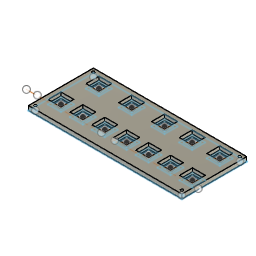
keyboard-holder (Autodesk Fusion 360 design; units mm, degrees)
Autodesk Fusion 360 part; units mm, degrees
sketch "Sketch1" plane through (0, 0, 0) normal (0, 0, 1) x (1, 0, 0)
  line L0 (-23.9041, 0) -> (63.45, 0) construction
  line L1 (78.95, 0) -> (176.0959, 0) construction
  line L2 (-1.45, -20) -> (177.05, -20)
  line L3 (177.05, -20) -> (177.05, 55.5)
  line L4 (177.05, 55.5) -> (-1.45, 55.5)
  line L5 (-1.45, 55.5) -> (-1.45, -20)
  line L6 (6.3, 0) -> (16.3, 0)
  line L7 (16.3, 0) -> (16.3, 10)
  line L8 (16.3, 10) -> (6.3, 10)
  line L9 (6.3, 10) -> (6.3, 0)
  line L10 (31.8, 0) -> (41.8, 0)
  line L11 (41.8, 0) -> (41.8, 10)
  line L12 (41.8, 10) -> (31.8, 10)
  line L13 (31.8, 10) -> (31.8, 0)
  line L14 (57.3, 0) -> (67.3, 0)
  line L15 (67.3, 0) -> (67.3, 10)
  line L16 (67.3, 10) -> (57.3, 10)
  line L17 (57.3, 10) -> (57.3, 0)
  line L18 (82.8, 0) -> (92.8, 0)
  line L19 (92.8, 0) -> (92.8, 10)
  line L20 (92.8, 10) -> (82.8, 10)
  line L21 (82.8, 10) -> (82.8, 0)
  line L22 (108.3, 0) -> (118.3, 0)
  line L23 (118.3, 0) -> (118.3, 10)
  line L24 (118.3, 10) -> (108.3, 10)
  line L25 (108.3, 10) -> (108.3, 0)
  line L26 (133.8, 0) -> (143.8, 0)
  line L27 (143.8, 0) -> (143.8, 10)
  line L28 (143.8, 10) -> (133.8, 10)
  line L29 (133.8, 10) -> (133.8, 0)
  line L30 (159.3, 0) -> (169.3, 0)
  line L31 (169.3, 0) -> (169.3, 10)
  line L32 (169.3, 10) -> (159.3, 10)
  line L33 (159.3, 10) -> (159.3, 0)
  line L34 (12.45, 48) -> (22.45, 48)
  line L35 (22.45, 48) -> (22.45, 38)
  line L36 (22.45, 38) -> (12.45, 38)
  line L37 (12.45, 38) -> (12.45, 48)
  line L38 (50.65, 48) -> (60.65, 48)
  line L39 (60.65, 48) -> (60.65, 38)
  line L40 (60.65, 38) -> (50.65, 38)
  line L41 (50.65, 38) -> (50.65, 48)
  line L42 (88.85, 48) -> (98.85, 48)
  line L43 (98.85, 48) -> (98.85, 38)
  line L44 (98.85, 38) -> (88.85, 38)
  line L45 (88.85, 38) -> (88.85, 48)
  line L46 (121, 48) -> (131, 48)
  line L47 (131, 48) -> (131, 38)
  line L48 (131, 38) -> (121, 38)
  line L49 (121, 38) -> (121, 48)
  line L50 (153.15, 48) -> (163.15, 48)
  line L51 (163.15, 48) -> (163.15, 38)
  line L52 (163.15, 38) -> (153.15, 38)
  line L53 (153.15, 38) -> (153.15, 48)
  line L54 (9.95, 50.5) -> (24.95, 50.5)
  line L55 (24.95, 50.5) -> (24.95, 35.5)
  line L56 (24.95, 35.5) -> (9.95, 35.5)
  line L57 (9.95, 35.5) -> (9.95, 50.5)
  line L58 (9.95, 50.5) -> (24.95, 35.5) construction
  line L59 (24.95, 50.5) -> (9.95, 35.5) construction
  line L60 (48.15, 50.5) -> (63.15, 50.5)
  line L61 (63.15, 50.5) -> (63.15, 35.5)
  line L62 (63.15, 35.5) -> (48.15, 35.5)
  line L63 (48.15, 35.5) -> (48.15, 50.5)
  line L64 (48.15, 50.5) -> (63.15, 35.5) construction
  line L65 (63.15, 50.5) -> (48.15, 35.5) construction
  line L66 (86.35, 50.5) -> (101.35, 50.5)
  line L67 (101.35, 50.5) -> (101.35, 35.5)
  line L68 (101.35, 35.5) -> (86.35, 35.5)
  line L69 (86.35, 35.5) -> (86.35, 50.5)
  line L70 (86.35, 50.5) -> (101.35, 35.5) construction
  line L71 (101.35, 50.5) -> (86.35, 35.5) construction
  line L72 (118.5, 50.5) -> (133.5, 50.5)
  line L73 (133.5, 50.5) -> (133.5, 35.5)
  line L74 (133.5, 35.5) -> (118.5, 35.5)
  line L75 (118.5, 35.5) -> (118.5, 50.5)
  line L76 (118.5, 50.5) -> (133.5, 35.5) construction
  line L77 (133.5, 50.5) -> (118.5, 35.5) construction
  line L78 (150.65, 50.5) -> (165.65, 50.5)
  line L79 (165.65, 50.5) -> (165.65, 35.5)
  line L80 (165.65, 35.5) -> (150.65, 35.5)
  line L81 (150.65, 35.5) -> (150.65, 50.5)
  line L82 (150.65, 50.5) -> (165.65, 35.5) construction
  line L83 (165.65, 50.5) -> (150.65, 35.5) construction
  line L84 (3.8, 12.5) -> (18.8, 12.5)
  line L85 (18.8, 12.5) -> (18.8, -2.5)
  line L86 (18.8, -2.5) -> (3.8, -2.5)
  line L87 (3.8, -2.5) -> (3.8, 12.5)
  line L88 (3.8, 12.5) -> (18.8, -2.5) construction
  line L89 (18.8, 12.5) -> (3.8, -2.5) construction
  line L90 (29.3, 12.5) -> (44.3, 12.5)
  line L91 (44.3, 12.5) -> (44.3, -2.5)
  line L92 (44.3, -2.5) -> (29.3, -2.5)
  line L93 (29.3, -2.5) -> (29.3, 12.5)
  line L94 (29.3, 12.5) -> (44.3, -2.5) construction
  line L95 (44.3, 12.5) -> (29.3, -2.5) construction
  line L96 (54.8, 12.5) -> (69.8, 12.5)
  line L97 (69.8, 12.5) -> (69.8, -2.5)
  line L98 (69.8, -2.5) -> (54.8, -2.5)
  line L99 (54.8, -2.5) -> (54.8, 12.5)
  line L100 (54.8, 12.5) -> (69.8, -2.5) construction
  line L101 (69.8, 12.5) -> (54.8, -2.5) construction
  line L102 (80.3, 12.5) -> (95.3, 12.5)
  line L103 (95.3, 12.5) -> (95.3, -2.5)
  line L104 (95.3, -2.5) -> (80.3, -2.5)
  line L105 (80.3, -2.5) -> (80.3, 12.5)
  line L106 (80.3, 12.5) -> (95.3, -2.5) construction
  line L107 (95.3, 12.5) -> (80.3, -2.5) construction
  line L108 (105.8, 12.5) -> (120.8, 12.5)
  line L109 (120.8, 12.5) -> (120.8, -2.5)
  line L110 (120.8, -2.5) -> (105.8, -2.5)
  line L111 (105.8, -2.5) -> (105.8, 12.5)
  line L112 (105.8, 12.5) -> (120.8, -2.5) construction
  line L113 (120.8, 12.5) -> (105.8, -2.5) construction
  line L114 (131.3, 12.5) -> (146.3, 12.5)
  line L115 (146.3, 12.5) -> (146.3, -2.5)
  line L116 (146.3, -2.5) -> (131.3, -2.5)
  line L117 (131.3, -2.5) -> (131.3, 12.5)
  line L118 (131.3, 12.5) -> (146.3, -2.5) construction
  line L119 (146.3, 12.5) -> (131.3, -2.5) construction
  line L120 (156.8, 12.5) -> (171.8, 12.5)
  line L121 (171.8, 12.5) -> (171.8, -2.5)
  line L122 (171.8, -2.5) -> (156.8, -2.5)
  line L123 (156.8, -2.5) -> (156.8, 12.5)
  line L124 (156.8, 12.5) -> (171.8, -2.5) construction
  line L125 (171.8, 12.5) -> (156.8, -2.5) construction
  circle A0 centre (2.55, 51.5) radius 1.5
  circle A1 centre (2.55, -16) radius 1.5
  circle A2 centre (173.05, -16) radius 1.5
  circle A3 centre (173.05, 51.5) radius 1.5
  point P0 (-11.7503, 0.5527)
  point P1 (17.45, 43)
  point P2 (55.65, 43)
  point P3 (93.85, 43)
  point P4 (126, 43)
  point P5 (158.15, 43)
  point P6 (11.3, 5)
  point P7 (36.8, 5)
  point P8 (62.3, 5)
  point P9 (87.8, 5)
  point P10 (113.3, 5)
  point P11 (138.8, 5)
  point P12 (164.3, 5)
  dimension "d77" = 200
  dimension "d86" = 75.5
  dimension "d89" = 10
  dimension "d90" = 10
  dimension "d91" = 20
  dimension "d92" = 7.75
  dimension "d93" = 10
  dimension "d94" = 10
  dimension "d95" = 10
  dimension "d96" = 10
  dimension "d99" = 10
  dimension "d100" = 10
  dimension "d101" = 15.5
  dimension "d102" = 15.5
  dimension "d104" = 15.5
  dimension "d105" = 10
  dimension "d106" = 10
  dimension "d107" = 15.5
  dimension "d108" = 10
  dimension "d109" = 10
  dimension "d110" = 15.5
  dimension "d111" = 10
  dimension "d112" = 10
  dimension "d113" = 15.5
  dimension "d114" = 10
  dimension "d115" = 10
  dimension "d116" = 13.9
  dimension "d117" = 7.5
  dimension "d118" = 10
  dimension "d119" = 10
  dimension "d120" = 7.5
  dimension "d121" = 28.2
  dimension "d122" = 10
  dimension "d123" = 10
  dimension "d124" = 28.2
  dimension "d125" = 7.5
  dimension "d126" = 10
  dimension "d127" = 10
  dimension "d128" = 22.15
  dimension "d129" = 7.5
  dimension "d130" = 10
  dimension "d131" = 10
  dimension "d132" = 22.15
  dimension "d133" = 7.5
  dimension "d134" = 15
  dimension "d135" = 15
  dimension "d136" = 15
  dimension "d137" = 15
  dimension "d138" = 15
  dimension "d139" = 15
  dimension "d140" = 15
  dimension "d141" = 15
  dimension "d142" = 15
  dimension "d143" = 15
  dimension "d144" = 15
  dimension "d145" = 15
  dimension "d146" = 15
  dimension "d147" = 15
  dimension "d148" = 15
  dimension "d149" = 15
  dimension "d150" = 15
  dimension "d151" = 15
  dimension "d152" = 15
  dimension "d153" = 15
  dimension "d154" = 15
  dimension "d155" = 15
  dimension "d156" = 15
  dimension "d157" = 15
  dimension "d158" = 3
  dimension "d159" = 4
  dimension "d160" = 4
  dimension "d161" = 3
  dimension "d162" = 4
  dimension "d163" = 4
  dimension "d164" = 3
  dimension "d165" = 4
  dimension "d166" = 4
  dimension "d167" = 3
  dimension "d168" = 4
  dimension "d169" = 4
  dimension "d174" = 2.5
  dimension "d175" = 2.5
  dimension "d176" = 2.5
  dimension "d177" = 2.5
  dimension "d178" = 2.5
  dimension "d179" = 2.5
  dimension "d182" = 5.25
  dimension "d183" = 2.5
  dimension "d184" = 2.5
  dimension "d185" = 2.5
  dimension "d186" = 2.5
  dimension "d187" = 2.5
  dimension "d188" = 2.5
  dimension "d189" = 2.5
  dimension "d190" = 2.5
  dimension "d191" = 2.5
  dimension "d192" = 2.5
  dimension "d193" = 2.5
  constraint horizontal L2
  constraint vertical L3
  constraint horizontal L4
  constraint vertical L5
  constraint horizontal L6
  constraint vertical L7
  constraint horizontal L8
  constraint vertical L9
  constraint horizontal L10
  constraint vertical L11
  constraint horizontal L12
  constraint vertical L13
  constraint coincident L0 L10.start
  constraint horizontal L14
  constraint vertical L15
  constraint horizontal L16
  constraint vertical L17
  constraint coincident L0 L14.start
  constraint horizontal L18
  constraint vertical L19
  constraint horizontal L20
  constraint vertical L21
  constraint coincident L1 L18.start
  constraint horizontal L22
  constraint vertical L23
  constraint horizontal L24
  constraint vertical L25
  constraint coincident L1 L22.start
  constraint horizontal L26
  constraint vertical L27
  constraint horizontal L28
  constraint vertical L29
  constraint coincident L1 L26.start
  constraint horizontal L30
  constraint vertical L31
  constraint horizontal L32
  constraint vertical L33
  constraint coincident L1 L30.start
  constraint horizontal L34
  constraint vertical L35
  constraint horizontal L36
  constraint vertical L37
  constraint horizontal L38
  constraint vertical L39
  constraint horizontal L40
  constraint vertical L41
  constraint horizontal L42
  constraint vertical L43
  constraint horizontal L44
  constraint vertical L45
  constraint horizontal L46
  constraint vertical L47
  constraint horizontal L48
  constraint vertical L49
  constraint horizontal L50
  constraint vertical L51
  constraint horizontal L52
  constraint vertical L53
  constraint horizontal L54
  constraint perpendicular L54 L55
  constraint parallel L54 L56
  constraint parallel L55 L57
  constraint coincident L58 P1
  constraint coincident L59 P1
  constraint horizontal L60
  constraint perpendicular L60 L61
  constraint parallel L60 L62
  constraint parallel L61 L63
  constraint coincident L64 P2
  constraint coincident L65 P2
  constraint horizontal L66
  constraint perpendicular L66 L67
  constraint parallel L66 L68
  constraint parallel L67 L69
  constraint coincident L70 P3
  constraint coincident L71 P3
  constraint horizontal L72
  constraint perpendicular L72 L73
  constraint parallel L72 L74
  constraint parallel L73 L75
  constraint coincident L76 P4
  constraint coincident L77 P4
  constraint horizontal L78
  constraint perpendicular L78 L79
  constraint parallel L78 L80
  constraint parallel L79 L81
  constraint coincident L82 P5
  constraint coincident L83 P5
  constraint horizontal L84
  constraint perpendicular L84 L85
  constraint parallel L84 L86
  constraint parallel L85 L87
  constraint coincident L88 P6
  constraint coincident L89 P6
  constraint horizontal L90
  constraint perpendicular L90 L91
  constraint parallel L90 L92
  constraint parallel L91 L93
  constraint coincident L94 P7
  constraint coincident L95 P7
  constraint horizontal L96
  constraint perpendicular L96 L97
  constraint parallel L96 L98
  constraint parallel L97 L99
  constraint coincident L100 P8
  constraint coincident L101 P8
  constraint horizontal L102
  constraint perpendicular L102 L103
  constraint parallel L102 L104
  constraint parallel L103 L105
  constraint coincident L106 P9
  constraint coincident L107 P9
  constraint horizontal L108
  constraint perpendicular L108 L109
  constraint parallel L108 L110
  constraint parallel L109 L111
  constraint coincident L112 P10
  constraint coincident L113 P10
  constraint horizontal L114
  constraint perpendicular L114 L115
  constraint parallel L114 L116
  constraint parallel L115 L117
  constraint coincident L118 P11
  constraint coincident L119 P11
  constraint horizontal L120
  constraint perpendicular L120 L121
  constraint parallel L120 L122
  constraint parallel L121 L123
  constraint coincident L124 P12
  constraint coincident L125 P12
  measures "d77" distance of L0.start L1.end
  measures "d86" distance of L2.start L4.end
  measures "d89" distance of L6.start L6.end
  measures "d90" distance of L6.start L8.end
  measures "d91" distance of L2 L6
  measures "d92" distance of L5 L9
  measures "d93" distance of L10.start L10.end
  measures "d94" distance of L10.start L12.end
  measures "d95" distance of L14.start L14.end
  measures "d96" distance of L14.start L16.end
  measures "d99" distance of L18.start L18.end
  measures "d100" distance of L18.start L20.end
  measures "d101" distance of L7 L13
  measures "d102" distance of L11 L17
  measures "d104" distance of L15 L21
  measures "d105" distance of L22.start L22.end
  measures "d106" distance of L22.start L24.end
  measures "d107" distance of L19 L25
  measures "d108" distance of L26.start L28.end
  measures "d109" distance of L26.start L26.end
  measures "d110" distance of L23 L29
  measures "d111" distance of L30.start L30.end
  measures "d112" distance of L30.start L32.end
  measures "d113" distance of L27 L33
  measures "d114" distance of L34.start L34.end
  measures "d115" distance of L34.start L36.end
  measures "d116" distance of L5 L37
  measures "d117" distance of L4 L34
  measures "d118" distance of L38.start L38.end
  measures "d119" distance of L38.start L40.end
  measures "d120" distance of L4 L38
  measures "d121" distance of L35 L41
  measures "d122" distance of L42.start L42.end
  measures "d123" distance of L42.start L44.end
  measures "d124" distance of L39 L45
  measures "d125" distance of L4 L42
  measures "d126" distance of L46.start L46.end
  measures "d127" distance of L46.start L48.end
  measures "d128" distance of L43 L49
  measures "d129" distance of L4 L46
  measures "d130" distance of L50.start L50.end
  measures "d131" distance of L50.start L52.end
  measures "d132" distance of L47 L53
  measures "d133" distance of L4 L50
  measures "d134" distance of L55.end L56.end
  measures "d135" distance of L54.end L55.end
  measures "d136" distance of L61.end L62.end
  measures "d137" distance of L60.end L61.end
  measures "d138" distance of L67.end L68.end
  measures "d139" distance of L66.end L67.end
  measures "d140" distance of L73.end L74.end
  measures "d141" distance of L72.end L73.end
  measures "d142" distance of L79.end L80.end
  measures "d143" distance of L78.end L79.end
  measures "d144" distance of L85.end L86.end
  measures "d145" distance of L84.end L85.end
  measures "d146" distance of L91.end L92.end
  measures "d147" distance of L90.end L91.end
  measures "d148" distance of L97.end L98.end
  measures "d149" distance of L96.end L97.end
  measures "d150" distance of L103.end L104.end
  measures "d151" distance of L102.end L103.end
  measures "d152" distance of L109.end L110.end
  measures "d153" distance of L108.end L109.end
  measures "d154" distance of L115.end L116.end
  measures "d155" distance of L114.end L115.end
  measures "d156" distance of L121.end L122.end
  measures "d157" distance of L120.end L121.end
  measures "d158" diameter of A0
  measures "d159" distance of L5 A0.centre
  measures "d160" distance of L4 A0.centre
  measures "d161" diameter of A1
  measures "d162" distance of L5 A1.centre
  measures "d163" distance of L2 A1.centre
  measures "d164" diameter of A2
  measures "d165" distance of L3 A2.centre
  measures "d166" distance of L2 A2.centre
  measures "d167" diameter of A3
  measures "d168" distance of L4 A3.centre
  measures "d169" distance of L3 A3.centre
  measures "d174" distance of L13 L93
  measures "d175" distance of L17 L99
  measures "d176" distance of L21 L105
  measures "d177" distance of L25 L111
  measures "d178" distance of L29 L117
  measures "d179" distance of L33 L123
  measures "d182" distance of L3 L121
  measures "d183" distance of L36 L56
  measures "d184" distance of L40 L62
  measures "d185" distance of L44 L68
  measures "d186" distance of L48 L74
  measures "d187" distance of L52 L80
  measures "d188" distance of L41 L63
  measures "d189" distance of L45 L69
  measures "d190" distance of L49 L75
  measures "d191" distance of L53 L81
  measures "d192" distance of L37 L57
  measures "d193" distance of L9 L87
extrude "Extrude1" add sketch "Sketch1" along normal blind 1 contours L54 L55 L56 L57 | L60 L61 L62 L63 | L66 L67 L68 L69 | L72 L73 L74 L75 | L78 L79 L80 L81 | L84 L85 L86 L87 | L90 L91 L92 L93 | L96 L97 L98 L99 | L102 L103 L104 L105 | L108 L109 L110 L111 | L114 L115 L116 L117 | L120 L121 L122 L123 makes body 1 at (140.4667, 11.6667, 0) makes body 2 at (89.4667, 11.6667, 0) makes body 3 at (12.9667, -1.6667, 0) makes body 4 at (35.1333, 11.6667, 0) makes body 5 at (95.5167, 36.3333, 0) makes body 6 at (151.4833, 41.3333, 0) makes body 7 at (119.3333, 41.3333, 0) makes body 8 at (60.6333, -1.6667, 0) makes body 9 at (24.1167, 44.6667, 0) makes body 10 at (57.3167, 49.6667, 0) makes body 11 at (114.9667, -1.6667, 0) makes body 12 at (162.6333, 11.6667, 0)
extrude "Extrude2" add sketch "Sketch1" along normal blind 5 contours L2 L3 L4 L5 bodies 1 2 3 4 5 6 7 8 9 10 11 12
